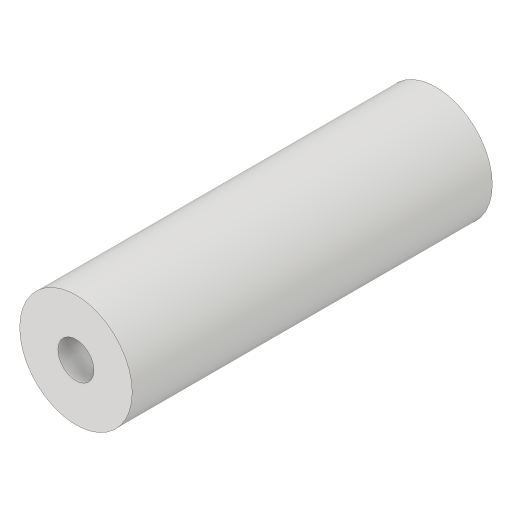
# Autodesk Inventor part: Gear_8T_Connect
Saved by Autodesk Inventor 2023.2 (Build 272271000, 271)
## iProperties
Created: 2021-07-28
Part Number: Gear_8T_Connect
Material: LCP 플라스틱
Document SubType Name: Modeling
Designer: user
Density: 1.626 g/cm^3
Appearance: 매끄러움 - 흰색
Mass: 1.80161 g
Surface Area: 10.5204 cm^2
Volume: 1.108 cm^3
Author: user
Autodesk Inventor part; units mm, degrees
ref_plane "YZ Plane" through (0, 0, 0) normal (1, 0, 0) x (0, 1, 0)
ref_plane "XZ Plane" through (0, 0, 0) normal (0, 1, 0) x (-1, 0, 0)
ref_plane "XY Plane" through (0, 0, 0) normal (0, 0, 1) x (1, 0, 0)
sketch "스케치1" plane through (0, 0, 0) normal (0, 0, 1) x (1, 0, 0)
  circle A0 centre (0, 0) radius 1.6
  circle A1 centre (0, 0) radius 5
  dimension "d0" = 3.2
  dimension "d1" = 10
  constraints: 2 centre point, 2 coincident
  measures "d0" diameter of A0
  measures "d1" diameter of A1
extrude "돌출1" add sketch "스케치1" along normal blind 32
